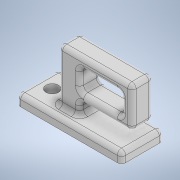
# Autodesk Inventor part: cable_holder
Saved by Autodesk Inventor 2021.4 (Build 254397000, 397)
## iProperties
Created: 2023-07-27
Part Number: cable_holder
Material: 一般
Document SubType Name: Modeling
Designer: ryusei
Density: 1 g/cm^3
Appearance: 既定
Author: ryusei
Autodesk Inventor part; units mm, degrees
ref_plane "YZ Plane" through (0, 0, 0) normal (1, 0, 0) x (0, 1, 0)
ref_plane "XZ Plane" through (0, 0, 0) normal (0, 1, 0) x (-1, 0, 0)
ref_plane "XY Plane" through (0, 0, 0) normal (0, 0, 1) x (1, 0, 0)
sketch "スケッチ1" plane through (0, 0, 0) normal (0, 1, 0) x (-1, 0, 0)
  line L0 (25, 10) -> (-25, 10)
  line L1 (-25, 10) -> (-25, -10)
  line L2 (-25, -10) -> (25, -10)
  line L3 (25, -10) -> (25, 10)
  line L4 (25, 10) -> (-25, -10) construction
  line L5 (-25, 10) -> (25, -10) construction
  point P0 (0, 0)
  dimension "d0" = 20
  dimension "d1" = 50
  constraints: 12 end point, 2 midpoint, 2 parallel, 1 horizontal, 1 perpendicular
  measures "d0" distance of L0.end L1.end
  measures "d1" distance of L1.end L2.end
extrude "押し出し1" add sketch "スケッチ1" along normal blind 5
sketch "スケッチ4" plane through (0, 5, 0) normal (0, 1, 0) x (1, 0, 0)
  line L0 (-25, -10) -> (25, -10) projected
  line L1 (-25, 10) -> (-25, -10) projected
  line L2 (25, -10) -> (25, 10) projected
  point P0 (0, 0)
  point P1 (-18, 0)
  dimension "d17" = 10
  dimension "d18" = 7
  measures "d17" distance from line of L0 point (-18, 0)
  measures "d18" distance from line of L1 point (-18, 0)
hole "穴2" at (-18, 5, 0) direction (0, -1, 0) diameter 6 end through all
sketch "スケッチ5" plane through (0, 5, 0) normal (0, 1, 0) x (1, 0, 0)
  line L0 (-10, 5) -> (25, 5)
  line L1 (25, 5) -> (25, -5)
  line L2 (25, -5) -> (-10, -5)
  line L3 (-10, -5) -> (-10, 5)
  line L4 (-25, 10) -> (-25, -10) projected
  point P0 (0, 0)
  dimension "d30" = 10
  dimension "d31" = 35
  dimension "d32" = 5
  dimension "d45" = 15
  constraints: 8 end point, 2 parallel, 1 horizontal, 1 perpendicular
  measures "d30" distance of L2.end L0.start
  measures "d31" distance of L0.start L0.end
  measures "d32" distance from line of point (0, 0) L0
  measures "d45" distance between parallel lines of L4 L3
extrude "押し出し3" add sketch "スケッチ5" along normal blind 25
sketch "スケッチ6" plane through (0, 0, 0) normal (0, -1, 0) x (1, 0, 0)
  line L0 (-5, 2.75) -> (5, 2.75)
  line L1 (5, 2.75) -> (5, -2.75)
  line L2 (5, -2.75) -> (-5, -2.75)
  line L3 (-5, -2.75) -> (-5, 2.75)
  line L4 (-5, 2.75) -> (5, -2.75) construction
  line L5 (5, 2.75) -> (-5, -2.75) construction
  point P0 (0, 0)
  dimension "d35" = 10
  dimension "d36" = 5.5
  constraints: 12 end point, 2 midpoint, 2 parallel, 1 horizontal, 1 perpendicular
  measures "d35" distance of L0.start L0.end
  measures "d36" distance of L0.end L1.end
extrude "押し出し4" add sketch "スケッチ6" along normal blind 3
sketch "スケッチ8" plane through (-10, 30, 5) normal (0, 0, 1) x (1, 0, 0)
  line L0 (10, -19) -> (35, -19)
  line L1 (35, -19) -> (35, -25)
  line L2 (35, -25) -> (10, -25)
  line L3 (10, -25) -> (10, -19)
  line L4 (30, -5) -> (30, -20) projected
  line L5 (35, -25) -> (35, 0) projected
  line L6 (-15, -25) -> (35, -25) projected
  point P0 (10, -30)
  dimension "d47" = 0
  dimension "d48" = 0
  dimension "d49" = 6
  dimension "d58" = 25
  constraints: 8 end point, 2 parallel, 1 horizontal, 1 perpendicular, 1 other
  measures "d47" distance between parallel lines of L5 L1
  measures "d48" vertical extent of L2
  measures "d49" distance between parallel lines of L2 L0
  measures "d58" distance of L0.start L0.end
extrude "押し出し6" cut sketch "スケッチ8" against normal through all
sketch "スケッチ9" plane through (-10, 30, 5) normal (0, 0, 1) x (1, 0, 0)
  line L0 (30, -5) -> (10, -5)
  line L1 (10, -5) -> (10, -15)
  line L2 (10, -15) -> (30, -15)
  line L3 (30, -15) -> (30, -5)
  line L4 (0, 0) -> (35, 0) projected
  line L5 (35, -19) -> (35, 0) projected
  point P0 (10, -30)
  dimension "d52" = 5
  dimension "d53" = 5
  dimension "d54" = 20
  dimension "d55" = 10
  constraints: 8 end point, 2 parallel, 1 horizontal, 1 perpendicular
  measures "d52" distance between parallel lines of L4 L0
  measures "d53" distance between parallel lines of L5 L3
  measures "d54" distance of L1.end L2.end
  measures "d55" distance of L2.end L0.start
extrude "押し出し7" cut sketch "スケッチ9" against normal through all
fillet "フィレット2" radius 2 38 edges at (-10, 17.5, 5) (10, 15, 5) (10, 15, -5) (12.5, 11, -5) (-10, 17.5, -5) (0, 11, 0) (0, 8, -5) (12.5, 11, 5) (0, 8, 5) (25, 20.5, 5) (25, 20.5, -5) (25, 11, 0) (20, 15, 0) (20, 20, 5) (20, 20, -5) (0, 15, 0) (-10, 30, 0) (0, 25, 0) (0, 20, -5) (7.5, 30, 5) (7.5, 30, -5) (10, 25, -5) (10, 25, 5) (0, 20, 5) (25, 30, 0) (20, 25, 0) (0, 5, 0) (-5, 5, 5) (-10, 5, 0) (-5, 5, -5) (0, 5, -10) (-25, 5, 0) (0, 5, 10) (-25, 2.5, -10) (-25, 2.5, 10) (25, 2.5, -10) (25, 5, 0) (25, 2.5, 10)
